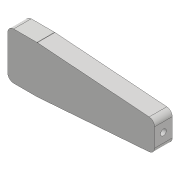
# Autodesk Inventor part: Switch_Extend
Saved by Autodesk Inventor 2018 (Build 220112000, 112)
## iProperties
Created: 2019-11-23
Part Number: Switch_Extend
Material: Generic
Document SubType Name: Modeling
Designer: Clevo
Density: 1 g/cm^3
Appearance: Default
Author: Clevo
Autodesk Inventor part; units mm, degrees
ref_plane "YZ Plane" through (0, 0, 0) normal (1, 0, 0) x (0, 1, 0)
ref_plane "XZ Plane" through (0, 0, 0) normal (0, 1, 0) x (-1, 0, 0)
ref_plane "XY Plane" through (0, 0, 0) normal (0, 0, 1) x (1, 0, 0)
sketch "Sketch1" plane through (0, 0, 0) normal (0, 1, 0) x (-1, 0, 0)
  line L0 (-12.5, -4) -> (12.5, -4)
  line L1 (12.5, -4) -> (12.5, 4)
  line L2 (12.5, 4) -> (-12.5, 4)
  line L3 (-12.5, 4) -> (-12.5, -4)
  line L4 (-12.5, -4) -> (12.5, 4) construction
  line L5 (12.5, -4) -> (-12.5, 4) construction
  point P0 (0, 0)
  dimension "d0" = 8
  dimension "d1" = 25
  constraints: 12 end point, 2 midpoint, 2 parallel, 1 horizontal, 1 perpendicular
  measures "d0" distance of L0.end L1.end
  measures "d1" distance of L1.end L2.end
extrude "Extrusion1" add sketch "Sketch1" along normal blind 3
sketch "Sketch2" plane through (0, 3, 0) normal (0, 1, 0) x (1, 0, 0)
  line L0 (12.5, 4) -> (-12.5, 4) projected
  line L1 (-12.5, 4) -> (-12.5, -4) projected
  line L2 (-12.5, -4) -> (12.5, -4) projected
  line L3 (12.5, -4) -> (12.5, 4) projected
  line L4 (-12.5, -4) -> (12.5, -4) projected
  line L5 (-7.5, -4) -> (12.5, -2.5)
  line L6 (12.5, -4) -> (12.5, 4) projected
  point P0 (0, 0)
  dimension "d4" = 20
  dimension "d5" = 1.5
  constraints: 2 end point, 2 point on line
  measures "d4" distance from line of L3 L5.start
  measures "d5" distance from line of L2 L5.end
extrude "Extrusion2" cut sketch "Sketch2" against normal through all contours L3 L2 L5
mirror "Mirror1" about plane through (0, 0, 0) normal (0, 0, 1) of "Extrusion2"
fillet "Fillet1" radius 1 6 edges at (-12.5, 1.5, 4) (-12.5, 1.5, -4) (-7.5, 1.5, -4) (-7.5, 1.5, 4) (12.5, 1.5, 2.5) (12.5, 1.5, -2.5)
sketch "Sketch3" plane through (12.5, 0, 1.5722) normal (1, 0, 0) x (0, 0, -1)
  line L0 (3.1444, 3) -> (3.1444, 0) projected
  line L1 (0, 3) -> (3.1444, 3) projected
  line L2 (0, 0) -> (0, 3) projected
  line L3 (0, 0) -> (3.1444, 0) projected
  line L4 (3.1444, 3) -> (0, 3)
  line L5 (0, 3) -> (0, 0)
  line L6 (0, 0) -> (3.1444, 0)
  line L7 (3.1444, 0) -> (3.1444, 3)
  line L8 (3.1444, 3) -> (0, 0) construction
  line L9 (0, 3) -> (3.1444, 0) construction
  point P0 (1.5722, 0)
  point P1 (1.5722, 1.5)
  constraints: 12 end point, 2 midpoint, 2 parallel, 1 horizontal, 1 perpendicular
hole "Hole1" at (12.5, 1.5, 0) direction (-1, 0, 0) diameter 1 depth 8 tip angle 118
body "Solid1"
